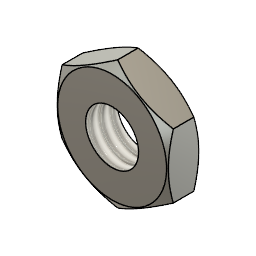
Cruiser Pedals v136 (Autodesk Fusion 360 archive; units mm, degrees)
design "Hexagon Nut BS 4183 - M4 Steel 6 Plain"
description: Hexagon Nut BS 4183 - M4
part number: HN BS 4183 - M4 Steel 6 Plain
Autodesk Fusion 360 part; units mm, degrees
sketch "Sketch1" plane through (0, 0, 0) normal (0, 1, 0) x (1, 0, 0)
  line L0 (0, 0) -> (0, -2)
  line L1 (-2, 0) -> (-3.43, 0)
  line L2 (-3.43, 0) -> (-4.0425, -0.3536)
  line L3 (-4.0425, -0.3536) -> (-4.0425, -1.6464)
  line L4 (-4.0425, -1.6464) -> (-3.43, -2)
  line L5 (-3.43, -2) -> (-2, -2)
  line L6 (-2, -2) -> (-2, 0)
  dimension "d121" = 4
  dimension "d122" = 30
  dimension "d123" = 30
  dimension "d125" = 6.86
  dimension "d128" = 8.085
  dimension "d152" = 2
  constraint vertical L0
  constraint coincident L0 L0.end
  constraint coincident origin L0
  constraint horizontal L1
  constraint perpendicular L1 L3
  constraint perpendicular L3 L5
  constraint perpendicular L5 L6
  constraint coincident L0.start L1
  constraint coincident L0.start origin
  constraint vertical L1.end L4.end
  constraint coincident L0.end L5
  measures "d122" angle of L1 L2
  measures "d123" angle of L4 L5
  measures "d152" distance of L1.start L5
revolve "Revolve1" add sketch "Sketch1" angle 360 about axis through (0, 0, 0) along (0, 0, 1)
sketch "Sketch8" plane through (0, 0, 2) normal (0, 0, 1) x (1, 0, 0)
  line L0 (0, 0) -> (-7, 0) construction
  line L1 (-3.5, -2.0228) -> (-3.5, 2.0228)
  circle A0 centre (0, 0) radius 2
  circle A1 centre (0, 0) radius 4.0425
  dimension "d114" = 3.5
  constraint horizontal L0
  constraint perpendicular L0 L1
  constraint midpoint L0 L1
  constraint coincident L0.start A0.centre
  constraint coincident L1.end A1
  measures "d114" distance of L0.start L1
extrude "Extrude5" cut sketch "Sketch8" against normal blind 2 contours L1 A1 picked at (-3.5875, 0.4927)
pattern_circular "C-Pattern2" count 6 over 360 about axis through (0, 0, 1.75) along (0, 0, 1) of "Extrude5"
thread "Thread3" "ISO Metric profile 4.0 M4x0.7 M4x0.7 6H" major diameter 4.1095 minor diameter 3.332 pitch 0.7 angle 60 resizes the face on face at (-1.9901, 0.1991, 1.3333)
equation "adsk_nheig = 2.00 mm"
equation "adsk_maxdia = 8.085 mm"
equation "adsk_nomdia = 4.00 mm"
equation "d89 = -adsk_nheig"
equation "adsk_waflat = 7.00 mm"
equation "d114 = adsk_waflat / 2"
equation "adsk_chamang1 = 30 deg"
equation "adsk_chamang2 = 30 deg"
equation "d121 = adsk_nomdia"
equation "d122 = adsk_chamang1"
equation "d123 = adsk_chamang2"
equation "d125 = adsk_beardia"
equation "d128 = adsk_maxdia"
equation "d147 = adsk_nheig"
equation "adsk_beardia = adsk_waflat * 0.98"
equation "d152 = adsk_nheig"

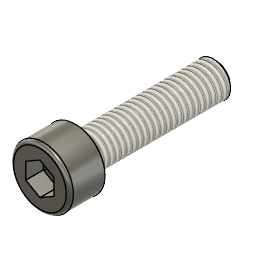
design "Broached Hexagon Socket Head Cap Screw ANSI B18.3.1M - M5x0.8 x 20 Steel Grade 2 Plain"
description: Broached Hexagon Socket Head Cap Screw ANSI B18.3.1M - M5x0.8 x 20
part number: BSHCS ANSI B18.3.1M - M5x0.8 x 20 Steel Grade 2 Plain
Autodesk Fusion 360 part; units mm, degrees
sketch "Sketch1" plane through (0, 0, 0) normal (0, 1, 0) x (1, 0, 0)
  line L0 (-2.5, 0) -> (-2.5, 20)
  line L1 (-2.5, 20) -> (0, 20)
  line L2 (0, 20) -> (0, -5)
  line L3 (-2.5, 0) -> (-4.25, 0)
  line L4 (-4.25, 0) -> (-4.25, -5)
  line L5 (-4.25, -5) -> (0, -5)
  dimension "d9" = 5
  dimension "d66" = 8.5
  dimension "d101" = 20
  dimension "d102" = 5
  constraint perpendicular L0 L1
  constraint collinear origin L1.end L2.end
  constraint perpendicular L0 L3
  constraint coincident origin L3
  constraint vertical L0
  constraint vertical L2
  constraint parallel L2 L4
  constraint coincident L2 L5.end
  constraint perpendicular L2 L5
  measures "d101" distance of origin L1
  measures "d102" distance of L3.end L5
revolve "Revolve1" add sketch "Sketch1" angle 360 about axis through (0, 0, -20) along (0, 0, 1)
ref_plane "WorkPlane1" through (0, 0, 5) normal (0, 0, 1) x (1, 0, 0)
sketch "Sketch6" plane through (0, 0, 5) normal (0, 0, 1) x (1, 0, 0)
  line L0 (-2, 0) -> (2, 0) construction
  line L1 (0, 0) -> (-2, 1.1547)
  line L2 (-2, -1.1547) -> (-2, 1.1547)
  line L3 (-2, -1.1547) -> (0, 0)
  dimension "d100" = 150
  dimension "d103" = 4
  constraint horizontal L0
  constraint midpoint L1.start L0
  constraint coincident L1.start L3.end
  constraint perpendicular L0 L2
  constraint midpoint L0.start L2
  constraint coincident L1.end L2.end
  measures "d100" angle of L0 L1
  measures "d103" distance of L0.end L2
extrude "Extrude1" cut sketch "Sketch6" against normal blind 2.5
pattern_circular "C-Pattern1" count 6 over 360 about axis through (0, 0, 1.75) along (0, 0, 1) of "Extrude1"
extrude "Extrude2" cut 1 faces at (0, -0.7698, 2.5) along direction (0, 0, -1) blind 2.5 draft -85
thread "Thread3" "ANSI Metric M Profile 5.0 M5x0.8 M5x0.8 4g6g" major diameter 4.901 minor diameter 4.007 pitch 0.8 angle 60 resizes the face on face at (-2.4969, 0.1246, -6.6667) from (0, 0, -1.4815) to (0, 0, -20)
fillet "Fillet4" radius 0.5 1 edges at (-3.9624, 1.5369, 5)
sketch "Sketch7" plane through (0, 0, 0) normal (0, 1, 0) x (1, 0, 0)
  line L0 (-2.55, 20) -> (-2.55, 19.5092)
  line L1 (-2.55, 19.5092) -> (-2.0092, 20)
  line L2 (0, 20) -> (0, -5)
  line L3 (-2.55, 20) -> (0, 20)
  dimension "d104" = 2.0092
  dimension "d105" = 2.55
  dimension "d106" = 0.4908
  constraint coincident L2.start L3.end
  constraint perpendicular L2 L3
  constraint coincident L1.end L3
  constraint perpendicular L0 L3
  measures "d104" distance of L1.end L2
  measures "d105" distance of L0 L2.start
  measures "d106" distance of L0.end L3
revolve "Revolve3" cut sketch "Sketch7" angle 360 about axis through (0, 0, 1.75) along (0, 0, 1)
equation "d9 = adsk_nomdia"
equation "adsk_nomlen = 20.00 mm"
equation "adsk_headh = 5.00 mm"
equation "adsk_headdia = 8.50 mm"
equation "adsk_nomdia = 5.00 mm"
equation "adsk_philwidth = 4.00 mm"
equation "d31 = -adsk_phildepth"
equation "adsk_phildepth = 2.50 mm"
equation "d66 = adsk_headdia"
equation "d71 = adsk_headh"
equation "d76 = -adsk_phildepth"
equation "adsk_thrlen = 18.51848 mm"
equation "d86 = adsk_nomdia * 0.1"
equation "adsk_startlen = 0.49076 mm"
equation "adsk_endpointdia = 4.01848 mm"
equation "d101 = adsk_nomlen"
equation "d102 = adsk_headh"
equation "d103 = adsk_philwidth"
equation "d104 = adsk_endpointdia / 2"
equation "d105 = adsk_nomdia * 0.51"
equation "d106 = adsk_startlen"
equation "d108 = min(adsk_thrlen; adsk_nomlen - 0.001 mm)"

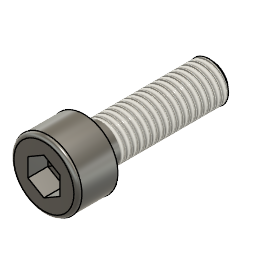
design "Broached Hexagon Socket Head Cap Screw ANSI B18.3.1M - M5x0.8 x 16 Steel Grade 2 Plain"
description: Broached Hexagon Socket Head Cap Screw ANSI B18.3.1M - M5x0.8 x 16
part number: BSHCS ANSI B18.3.1M - M5x0.8 x 16 Steel Grade 2 Plain
Autodesk Fusion 360 part; units mm, degrees
sketch "Sketch1" plane through (0, 0, 0) normal (0, 1, 0) x (1, 0, 0)
  line L0 (-2.5, 0) -> (-2.5, 16)
  line L1 (-2.5, 16) -> (0, 16)
  line L2 (0, 16) -> (0, -5)
  line L3 (-2.5, 0) -> (-4.25, 0)
  line L4 (-4.25, 0) -> (-4.25, -5)
  line L5 (-4.25, -5) -> (0, -5)
  dimension "d9" = 5
  dimension "d66" = 8.5
  dimension "d101" = 16
  dimension "d102" = 5
  constraint perpendicular L0 L1
  constraint collinear origin L1.end L2.end
  constraint perpendicular L0 L3
  constraint coincident origin L3
  constraint vertical L0
  constraint vertical L2
  constraint parallel L2 L4
  constraint coincident L2 L5.end
  constraint perpendicular L2 L5
  measures "d101" distance of origin L1
  measures "d102" distance of L3.end L5
revolve "Revolve1" add sketch "Sketch1" angle 360 about axis through (0, 0, -16) along (0, 0, 1)
ref_plane "WorkPlane1" through (0, 0, 5) normal (0, 0, 1) x (1, 0, 0)
sketch "Sketch6" plane through (0, 0, 5) normal (0, 0, 1) x (1, 0, 0)
  line L0 (-2, 0) -> (2, 0) construction
  line L1 (0, 0) -> (-2, 1.1547)
  line L2 (-2, -1.1547) -> (-2, 1.1547)
  line L3 (-2, -1.1547) -> (0, 0)
  dimension "d100" = 150
  dimension "d103" = 4
  constraint horizontal L0
  constraint midpoint L1.start L0
  constraint coincident L1.start L3.end
  constraint perpendicular L0 L2
  constraint midpoint L0.start L2
  constraint coincident L1.end L2.end
  measures "d100" angle of L0 L1
  measures "d103" distance of L0.end L2
extrude "Extrude1" cut sketch "Sketch6" against normal blind 2.5
pattern_circular "C-Pattern1" count 6 over 360 about axis through (0, 0, 1.75) along (0, 0, 1) of "Extrude1"
extrude "Extrude2" cut 1 faces at (-0.6667, 0.3849, 2.5) along direction (0, 0, -1) blind 2.5 draft -85
thread "Thread3" "ANSI Metric M Profile 5.0 M5x0.8 M5x0.8 4g6g" major diameter 4.901 minor diameter 4.007 pitch 0.8 angle 60 resizes the face on face at (-2.4969, 0.1246, -5.3333) from (0, 0, -2.0908) to (0, 0, -16)
fillet "Fillet4" radius 0.5 1 edges at (-3.9624, 1.5369, 5)
sketch "Sketch7" plane through (0, 0, 0) normal (0, 1, 0) x (1, 0, 0)
  line L0 (-2.55, 16) -> (-2.55, 15.5092)
  line L1 (-2.55, 15.5092) -> (-2.0092, 16)
  line L2 (0, 16) -> (0, -5)
  line L3 (-2.55, 16) -> (0, 16)
  dimension "d104" = 2.0092
  dimension "d105" = 2.55
  dimension "d106" = 0.4908
  constraint coincident L2.start L3.end
  constraint perpendicular L2 L3
  constraint coincident L1.end L3
  constraint perpendicular L0 L3
  measures "d104" distance of L1.end L2
  measures "d105" distance of L0 L2.start
  measures "d106" distance of L0.end L3
revolve "Revolve3" cut sketch "Sketch7" angle 360 about axis through (0, 0, 1.75) along (0, 0, 1)
equation "d9 = adsk_nomdia"
equation "adsk_nomlen = 16.00 mm"
equation "adsk_headh = 5.00 mm"
equation "adsk_headdia = 8.50 mm"
equation "adsk_nomdia = 5.00 mm"
equation "adsk_philwidth = 4.00 mm"
equation "d31 = -adsk_phildepth"
equation "adsk_phildepth = 2.50 mm"
equation "d66 = adsk_headdia"
equation "d71 = adsk_headh"
equation "d76 = -adsk_phildepth"
equation "adsk_thrlen = 13.90924 mm"
equation "d86 = adsk_nomdia * 0.1"
equation "adsk_startlen = 0.49076 mm"
equation "adsk_endpointdia = 4.01848 mm"
equation "d101 = adsk_nomlen"
equation "d102 = adsk_headh"
equation "d103 = adsk_philwidth"
equation "d104 = adsk_endpointdia / 2"
equation "d105 = adsk_nomdia * 0.51"
equation "d106 = adsk_startlen"
equation "d108 = min(adsk_thrlen; adsk_nomlen - 0.001 mm)"

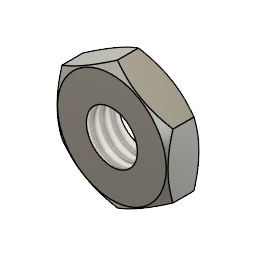
design "Hexagon Nut BS 4183 - M3 Steel 6 Plain"
description: Hexagon Nut BS 4183 - M3
part number: HN BS 4183 - M3 Steel 6 Plain
Autodesk Fusion 360 part; units mm, degrees
sketch "Sketch1" plane through (0, 0, 0) normal (0, 1, 0) x (1, 0, 0)
  line L0 (0, 0) -> (0, -1.6)
  line L1 (-1.5, 0) -> (-2.695, 0)
  line L2 (-2.695, 0) -> (-3.1763, -0.2778)
  line L3 (-3.1763, -0.2778) -> (-3.1763, -1.3222)
  line L4 (-3.1763, -1.3222) -> (-2.695, -1.6)
  line L5 (-2.695, -1.6) -> (-1.5, -1.6)
  line L6 (-1.5, -1.6) -> (-1.5, 0)
  dimension "d121" = 3
  dimension "d122" = 30
  dimension "d123" = 30
  dimension "d125" = 5.39
  dimension "d128" = 6.3525
  dimension "d152" = 1.6
  constraint vertical L0
  constraint coincident L0 L0.end
  constraint coincident origin L0
  constraint horizontal L1
  constraint perpendicular L1 L3
  constraint perpendicular L3 L5
  constraint perpendicular L5 L6
  constraint coincident L0.start L1
  constraint coincident L0.start origin
  constraint vertical L1.end L4.end
  constraint coincident L0.end L5
  measures "d122" angle of L1 L2
  measures "d123" angle of L4 L5
  measures "d152" distance of L1.start L5
revolve "Revolve1" add sketch "Sketch1" angle 360 about axis through (0, 0, 0) along (0, 0, 1)
sketch "Sketch8" plane through (0, 0, 1.6) normal (0, 0, 1) x (1, 0, 0)
  line L0 (0, 0) -> (-5.5, 0) construction
  line L1 (-2.75, -1.5894) -> (-2.75, 1.5894)
  circle A0 centre (0, 0) radius 1.5
  circle A1 centre (0, 0) radius 3.1763
  dimension "d114" = 2.75
  constraint horizontal L0
  constraint perpendicular L0 L1
  constraint midpoint L0 L1
  constraint coincident L0.start A0.centre
  constraint coincident L1.end A1
  measures "d114" distance of L0.start L1
extrude "Extrude5" cut sketch "Sketch8" against normal blind 1.6 contours L1 A1 picked at (-2.8188, 0.3871)
pattern_circular "C-Pattern2" count 6 over 360 about axis through (0, 0, 1.75) along (0, 0, 1) of "Extrude5"
thread "Thread3" "ISO Metric profile 3.0 M3x0.5 M3x0.5 6H" major diameter 3.086 minor diameter 2.529 pitch 0.5 angle 60 resizes the face on face at (-1.4981, 0.0748, 1.0667)
equation "adsk_nheig = 1.60 mm"
equation "adsk_maxdia = 6.3525 mm"
equation "adsk_nomdia = 3.00 mm"
equation "d89 = -adsk_nheig"
equation "adsk_waflat = 5.50 mm"
equation "d114 = adsk_waflat / 2"
equation "adsk_chamang1 = 30 deg"
equation "adsk_chamang2 = 30 deg"
equation "d121 = adsk_nomdia"
equation "d122 = adsk_chamang1"
equation "d123 = adsk_chamang2"
equation "d125 = adsk_beardia"
equation "d128 = adsk_maxdia"
equation "d147 = adsk_nheig"
equation "adsk_beardia = adsk_waflat * 0.98"
equation "d152 = adsk_nheig"

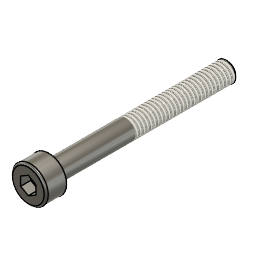
design "Broached Hexagon Socket Head Cap Screw ANSI B18.3.1M - M4x0.7 x 35 Steel Grade 2 Plain"
description: Broached Hexagon Socket Head Cap Screw ANSI B18.3.1M - M4x0.7 x 35
part number: BSHCS ANSI B18.3.1M - M4x0.7 x 35 Steel Grade 2 Plain
Autodesk Fusion 360 part; units mm, degrees
sketch "Sketch1" plane through (0, 0, 0) normal (0, 1, 0) x (1, 0, 0)
  line L0 (-2, 0) -> (-2, 35)
  line L1 (-2, 35) -> (0, 35)
  line L2 (0, 35) -> (0, -4)
  line L3 (-2, 0) -> (-3.5, 0)
  line L4 (-3.5, 0) -> (-3.5, -4)
  line L5 (-3.5, -4) -> (0, -4)
  dimension "d9" = 4
  dimension "d66" = 7
  dimension "d101" = 35
  dimension "d102" = 4
  constraint perpendicular L0 L1
  constraint collinear origin L1.end L2.end
  constraint perpendicular L0 L3
  constraint coincident origin L3
  constraint vertical L0
  constraint vertical L2
  constraint parallel L2 L4
  constraint coincident L2 L5.end
  constraint perpendicular L2 L5
  measures "d101" distance of origin L1
  measures "d102" distance of L3.end L5
revolve "Revolve1" add sketch "Sketch1" angle 360 about axis through (0, 0, -35) along (0, 0, 1)
ref_plane "WorkPlane1" through (0, 0, 4) normal (0, 0, 1) x (1, 0, 0)
sketch "Sketch6" plane through (0, 0, 4) normal (0, 0, 1) x (1, 0, 0)
  line L0 (-1.5, 0) -> (1.5, 0) construction
  line L1 (0, 0) -> (-1.5, 0.866)
  line L2 (-1.5, -0.866) -> (-1.5, 0.866)
  line L3 (-1.5, -0.866) -> (0, 0)
  dimension "d100" = 150
  dimension "d103" = 3
  constraint horizontal L0
  constraint midpoint L1.start L0
  constraint coincident L1.start L3.end
  constraint perpendicular L0 L2
  constraint midpoint L0.start L2
  constraint coincident L1.end L2.end
  measures "d100" angle of L0 L1
  measures "d103" distance of L0.end L2
extrude "Extrude1" cut sketch "Sketch6" against normal blind 2
pattern_circular "C-Pattern1" count 6 over 360 about axis through (0, 0, 1.75) along (0, 0, 1) of "Extrude1"
extrude "Extrude2" cut 1 faces at (0, -0.5774, 2) along direction (0, 0, -1) blind 2 draft -85
thread "Thread3" "ANSI Metric M Profile 4.0 M4x0.7 M4x0.7 4g6g" major diameter 3.908 minor diameter 3.128 pitch 0.7 angle 60 resizes the face on face at (-1.9901, 0.1991, -23.3333) from (0, 0, -15) to (0, 0, -35)
fillet "Fillet4" radius 0.4 1 edges at (-3.2631, 1.2657, 4)
sketch "Sketch7" plane through (0, 0, 0) normal (0, 1, 0) x (1, 0, 0)
  line L0 (-2.04, 35) -> (-2.04, 34.5706)
  line L1 (-2.04, 34.5706) -> (-1.5706, 35)
  line L2 (0, 35) -> (0, -4)
  line L3 (-2.04, 35) -> (0, 35)
  dimension "d104" = 1.5706
  dimension "d105" = 2.04
  dimension "d106" = 0.4294
  constraint coincident L2.start L3.end
  constraint perpendicular L2 L3
  constraint coincident L1.end L3
  constraint perpendicular L0 L3
  measures "d104" distance of L1.end L2
  measures "d105" distance of L0 L2.start
  measures "d106" distance of L0.end L3
revolve "Revolve3" cut sketch "Sketch7" angle 360 about axis through (0, 0, 1.75) along (0, 0, 1)
equation "d9 = adsk_nomdia"
equation "adsk_nomlen = 35.00 mm"
equation "adsk_headh = 4.00 mm"
equation "adsk_headdia = 7.00 mm"
equation "adsk_nomdia = 4.00 mm"
equation "adsk_philwidth = 3.00 mm"
equation "d31 = -adsk_phildepth"
equation "adsk_phildepth = 2.00 mm"
equation "d66 = adsk_headdia"
equation "d71 = adsk_headh"
equation "d76 = -adsk_phildepth"
equation "adsk_thrlen = 20.00 mm"
equation "d86 = adsk_nomdia * 0.1"
equation "adsk_startlen = 0.429415 mm"
equation "adsk_endpointdia = 3.14117 mm"
equation "d101 = adsk_nomlen"
equation "d102 = adsk_headh"
equation "d103 = adsk_philwidth"
equation "d104 = adsk_endpointdia / 2"
equation "d105 = adsk_nomdia * 0.51"
equation "d106 = adsk_startlen"
equation "d108 = min(adsk_thrlen; adsk_nomlen - 0.001 mm)"

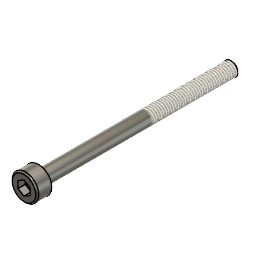
design "Broached Hexagon Socket Head Cap Screw ANSI B18.3.1M - M3x0.5 x 40 Steel Grade 2 Plain"
description: Broached Hexagon Socket Head Cap Screw ANSI B18.3.1M - M3x0.5 x 40
part number: BSHCS ANSI B18.3.1M - M3x0.5 x 40 Steel Grade 2 Plain
Autodesk Fusion 360 part; units mm, degrees
sketch "Sketch1" plane through (0, 0, 0) normal (0, 1, 0) x (1, 0, 0)
  line L0 (-1.5, 0) -> (-1.5, 40)
  line L1 (-1.5, 40) -> (0, 40)
  line L2 (0, 40) -> (0, -3)
  line L3 (-1.5, 0) -> (-2.75, 0)
  line L4 (-2.75, 0) -> (-2.75, -3)
  line L5 (-2.75, -3) -> (0, -3)
  dimension "d9" = 3
  dimension "d66" = 5.5
  dimension "d101" = 40
  dimension "d102" = 3
  constraint perpendicular L0 L1
  constraint collinear origin L1.end L2.end
  constraint perpendicular L0 L3
  constraint coincident origin L3
  constraint vertical L0
  constraint vertical L2
  constraint parallel L2 L4
  constraint coincident L2 L5.end
  constraint perpendicular L2 L5
  measures "d101" distance of origin L1
  measures "d102" distance of L3.end L5
revolve "Revolve1" add sketch "Sketch1" angle 360 about axis through (0, 0, -40) along (0, 0, 1)
ref_plane "WorkPlane1" through (0, 0, 3) normal (0, 0, 1) x (1, 0, 0)
sketch "Sketch6" plane through (0, 0, 3) normal (0, 0, 1) x (1, 0, 0)
  line L0 (-1.25, 0) -> (1.25, 0) construction
  line L1 (0, 0) -> (-1.25, 0.7217)
  line L2 (-1.25, -0.7217) -> (-1.25, 0.7217)
  line L3 (-1.25, -0.7217) -> (0, 0)
  dimension "d100" = 150
  dimension "d103" = 2.5
  constraint horizontal L0
  constraint midpoint L1.start L0
  constraint coincident L1.start L3.end
  constraint perpendicular L0 L2
  constraint midpoint L0.start L2
  constraint coincident L1.end L2.end
  measures "d100" angle of L0 L1
  measures "d103" distance of L0.end L2
extrude "Extrude1" cut sketch "Sketch6" against normal blind 1.5
pattern_circular "C-Pattern1" count 6 over 360 about axis through (0, 0, 1.75) along (0, 0, 1) of "Extrude1"
extrude "Extrude2" cut 1 faces at (0, -0.4811, 1.5) along direction (0, 0, -1) blind 1.5 draft -85
thread "Thread3" "ANSI Metric M Profile 3.0 M3x0.5 M3x0.5 4g6g" major diameter 2.927 minor diameter 2.369 pitch 0.5 angle 60 resizes the face on face at (-1.4981, 0.0748, -13.3333) from (0, 0, -22) to (0, 0, -40)
fillet "Fillet4" radius 0.3 1 edges at (-2.5639, 0.9944, 3)
sketch "Sketch7" plane through (0, 0, 0) normal (0, 1, 0) x (1, 0, 0)
  line L0 (-1.53, 40) -> (-1.53, 39.6933)
  line L1 (-1.53, 39.6933) -> (-1.1933, 40)
  line L2 (0, 40) -> (0, -3)
  line L3 (-1.53, 40) -> (0, 40)
  dimension "d104" = 1.1933
  dimension "d105" = 1.53
  dimension "d106" = 0.3067
  constraint coincident L2.start L3.end
  constraint perpendicular L2 L3
  constraint coincident L1.end L3
  constraint perpendicular L0 L3
  measures "d104" distance of L1.end L2
  measures "d105" distance of L0 L2.start
  measures "d106" distance of L0.end L3
revolve "Revolve3" cut sketch "Sketch7" angle 360 about axis through (0, 0, 1.75) along (0, 0, 1)
equation "d9 = adsk_nomdia"
equation "adsk_nomlen = 40.00 mm"
equation "adsk_headh = 3.00 mm"
equation "adsk_headdia = 5.50 mm"
equation "adsk_nomdia = 3.00 mm"
equation "adsk_philwidth = 2.50 mm"
equation "d31 = -adsk_phildepth"
equation "adsk_phildepth = 1.50 mm"
equation "d66 = adsk_headdia"
equation "d71 = adsk_headh"
equation "d76 = -adsk_phildepth"
equation "adsk_thrlen = 18.00 mm"
equation "d86 = adsk_nomdia * 0.1"
equation "adsk_startlen = 0.306725 mm"
equation "adsk_endpointdia = 2.38655 mm"
equation "d101 = adsk_nomlen"
equation "d102 = adsk_headh"
equation "d103 = adsk_philwidth"
equation "d104 = adsk_endpointdia / 2"
equation "d105 = adsk_nomdia * 0.51"
equation "d106 = adsk_startlen"
equation "d108 = min(adsk_thrlen; adsk_nomlen - 0.001 mm)"

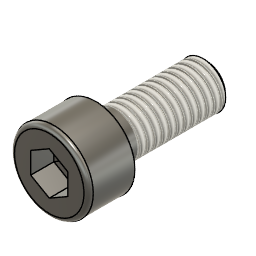
design "Broached Hexagon Socket Head Cap Screw ANSI B18.3.1M - M5x0.8 x 12 Steel Grade 2 Plain"
description: Broached Hexagon Socket Head Cap Screw ANSI B18.3.1M - M5x0.8 x 12
part number: BSHCS ANSI B18.3.1M - M5x0.8 x 12 Steel Grade 2 Plain
Autodesk Fusion 360 part; units mm, degrees
sketch "Sketch1" plane through (0, 0, 0) normal (0, 1, 0) x (1, 0, 0)
  line L0 (-2.5, 0) -> (-2.5, 12)
  line L1 (-2.5, 12) -> (0, 12)
  line L2 (0, 12) -> (0, -5)
  line L3 (-2.5, 0) -> (-4.25, 0)
  line L4 (-4.25, 0) -> (-4.25, -5)
  line L5 (-4.25, -5) -> (0, -5)
  dimension "d9" = 5
  dimension "d66" = 8.5
  dimension "d101" = 12
  dimension "d102" = 5
  constraint perpendicular L0 L1
  constraint collinear origin L1.end L2.end
  constraint perpendicular L0 L3
  constraint coincident origin L3
  constraint vertical L0
  constraint vertical L2
  constraint parallel L2 L4
  constraint coincident L2 L5.end
  constraint perpendicular L2 L5
  measures "d101" distance of origin L1
  measures "d102" distance of L3.end L5
revolve "Revolve1" add sketch "Sketch1" angle 360 about axis through (0, 0, -12) along (0, 0, 1)
ref_plane "WorkPlane1" through (0, 0, 5) normal (0, 0, 1) x (1, 0, 0)
sketch "Sketch6" plane through (0, 0, 5) normal (0, 0, 1) x (1, 0, 0)
  line L0 (-2, 0) -> (2, 0) construction
  line L1 (0, 0) -> (-2, 1.1547)
  line L2 (-2, -1.1547) -> (-2, 1.1547)
  line L3 (-2, -1.1547) -> (0, 0)
  dimension "d100" = 150
  dimension "d103" = 4
  constraint horizontal L0
  constraint midpoint L1.start L0
  constraint coincident L1.start L3.end
  constraint perpendicular L0 L2
  constraint midpoint L0.start L2
  constraint coincident L1.end L2.end
  measures "d100" angle of L0 L1
  measures "d103" distance of L0.end L2
extrude "Extrude1" cut sketch "Sketch6" against normal blind 2.5
pattern_circular "C-Pattern1" count 6 over 360 about axis through (0, 0, 1.75) along (0, 0, 1) of "Extrude1"
extrude "Extrude2" cut 1 faces at (0, 0.7698, 2.5) along direction (0, 0, -1) blind 2.5 draft -85
thread "Thread3" "ANSI Metric M Profile 5.0 M5x0.8 M5x0.8 4g6g" major diameter 4.901 minor diameter 4.007 pitch 0.8 angle 60 resizes the face on face at (-2.4969, 0.1246, -4) from (0, 0, -2.0908) to (0, 0, -12)
fillet "Fillet4" radius 0.5 1 edges at (-3.9624, 1.5369, 5)
sketch "Sketch7" plane through (0, 0, 0) normal (0, 1, 0) x (1, 0, 0)
  line L0 (-2.55, 12) -> (-2.55, 11.5092)
  line L1 (-2.55, 11.5092) -> (-2.0092, 12)
  line L2 (0, 12) -> (0, -5)
  line L3 (-2.55, 12) -> (0, 12)
  dimension "d104" = 2.0092
  dimension "d105" = 2.55
  dimension "d106" = 0.4908
  constraint coincident L2.start L3.end
  constraint perpendicular L2 L3
  constraint coincident L1.end L3
  constraint perpendicular L0 L3
  measures "d104" distance of L1.end L2
  measures "d105" distance of L0 L2.start
  measures "d106" distance of L0.end L3
revolve "Revolve3" cut sketch "Sketch7" angle 360 about axis through (0, 0, 1.75) along (0, 0, 1)
equation "d9 = adsk_nomdia"
equation "adsk_nomlen = 12.00 mm"
equation "adsk_headh = 5.00 mm"
equation "adsk_headdia = 8.50 mm"
equation "adsk_nomdia = 5.00 mm"
equation "adsk_philwidth = 4.00 mm"
equation "d31 = -adsk_phildepth"
equation "adsk_phildepth = 2.50 mm"
equation "d66 = adsk_headdia"
equation "d71 = adsk_headh"
equation "d76 = -adsk_phildepth"
equation "adsk_thrlen = 9.90924 mm"
equation "d86 = adsk_nomdia * 0.1"
equation "adsk_startlen = 0.49076 mm"
equation "adsk_endpointdia = 4.01848 mm"
equation "d101 = adsk_nomlen"
equation "d102 = adsk_headh"
equation "d103 = adsk_philwidth"
equation "d104 = adsk_endpointdia / 2"
equation "d105 = adsk_nomdia * 0.51"
equation "d106 = adsk_startlen"
equation "d108 = min(adsk_thrlen; adsk_nomlen - 0.001 mm)"

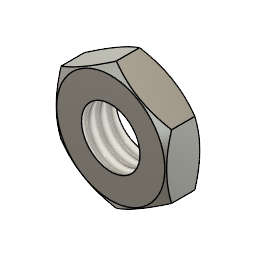
design "Hexagon Nut BS 4183 - M5 Steel 6 Plain"
description: Hexagon Nut BS 4183 - M5
part number: HN BS 4183 - M5 Steel 6 Plain
Autodesk Fusion 360 part; units mm, degrees
sketch "Sketch1" plane through (0, 0, 0) normal (0, 1, 0) x (1, 0, 0)
  line L0 (0, 0) -> (0, -2.5)
  line L1 (-2.5, 0) -> (-3.92, 0)
  line L2 (-3.92, 0) -> (-4.62, -0.4041)
  line L3 (-4.62, -0.4041) -> (-4.62, -2.0959)
  line L4 (-4.62, -2.0959) -> (-3.92, -2.5)
  line L5 (-3.92, -2.5) -> (-2.5, -2.5)
  line L6 (-2.5, -2.5) -> (-2.5, 0)
  dimension "d121" = 5
  dimension "d122" = 30
  dimension "d123" = 30
  dimension "d125" = 7.84
  dimension "d128" = 9.24
  dimension "d152" = 2.5
  constraint vertical L0
  constraint coincident L0 L0.end
  constraint coincident origin L0
  constraint horizontal L1
  constraint perpendicular L1 L3
  constraint perpendicular L3 L5
  constraint perpendicular L5 L6
  constraint coincident L0.start L1
  constraint coincident L0.start origin
  constraint vertical L1.end L4.end
  constraint coincident L0.end L5
  measures "d122" angle of L1 L2
  measures "d123" angle of L4 L5
  measures "d152" distance of L1.start L5
revolve "Revolve1" add sketch "Sketch1" angle 360 about axis through (0, 0, 0) along (0, 0, 1)
sketch "Sketch8" plane through (0, 0, 2.5) normal (0, 0, 1) x (1, 0, 0)
  line L0 (0, 0) -> (-8, 0) construction
  line L1 (-4, -2.3118) -> (-4, 2.3118)
  circle A0 centre (0, 0) radius 2.5
  circle A1 centre (0, 0) radius 4.62
  dimension "d114" = 4
  constraint horizontal L0
  constraint perpendicular L0 L1
  constraint midpoint L0 L1
  constraint coincident L0.start A0.centre
  constraint coincident L1.end A1
  measures "d114" distance of L0.start L1
extrude "Extrude5" cut sketch "Sketch8" against normal blind 2.5 contours L1 A1 picked at (-4.1, -0.5631)
pattern_circular "C-Pattern2" count 6 over 360 about axis through (0, 0, 1.75) along (0, 0, 1) of "Extrude5"
thread "Thread3" "ISO Metric profile 5.0 M5x0.8 M5x0.8 6H" major diameter 5.12 minor diameter 4.234 pitch 0.8 angle 60 resizes the face on face at (-2.4969, 0.1246, 1.6667)
equation "adsk_nheig = 2.50 mm"
equation "adsk_maxdia = 9.24 mm"
equation "adsk_nomdia = 5.00 mm"
equation "d89 = -adsk_nheig"
equation "adsk_waflat = 8.00 mm"
equation "d114 = adsk_waflat / 2"
equation "adsk_chamang1 = 30 deg"
equation "adsk_chamang2 = 30 deg"
equation "d121 = adsk_nomdia"
equation "d122 = adsk_chamang1"
equation "d123 = adsk_chamang2"
equation "d125 = adsk_beardia"
equation "d128 = adsk_maxdia"
equation "d147 = adsk_nheig"
equation "adsk_beardia = adsk_waflat * 0.98"
equation "d152 = adsk_nheig"
